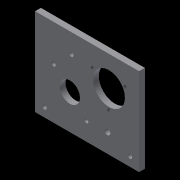
# Autodesk Inventor part: Main Outline
Saved by Autodesk Inventor 2014 SP1 (Build 180222100, 222)
## iProperties
Created: 2014-01-19
Part Number: Main Outline
Material: Generic
Document SubType Name: Modeling
Designer: Rauhul Varma
Density: 1 g/cm^3
Appearance: Default
Mass: 59.6414 g
Surface Area: 234.928 cm^2
Volume: 59.6414 cm^3
Author: Rauhul Varma
Autodesk Inventor part; units mm, degrees
ref_plane "YZ Plane" through (0, 0, 0) normal (1, 0, 0) x (0, 1, 0)
ref_plane "XZ Plane" through (0, 0, 0) normal (0, 1, 0) x (-1, 0, 0)
sketch "Sketch1" plane through (0, 0, 0) normal (0, 0, 1) x (1, 0, 0)
  line L0 (0, 0) -> (114.0582, 0)
  line L1 (114.0582, 0) -> (114.0582, 95.9104)
  line L2 (114.0582, 95.9104) -> (0, 95.9104)
  line L3 (0, 95.9104) -> (0, 0)
  line L4 (59.1, 17.1) -> (59.1, 59.1)
  line L5 (59.1, 59.1) -> (17.1, 59.1)
  line L6 (17.1, 59.1) -> (17.1, 17.1)
  line L7 (17.1, 17.1) -> (59.1, 17.1)
  line L8 (59.1, 17.1) -> (17.1, 59.1) construction
  line L9 (59.1, 59.1) -> (17.1, 17.1) construction
  circle A0 centre (38.1, 38.1) radius 38.1 construction
  circle A1 centre (38.1, 38.1) radius 20.2
  line L10 (45.4323, 38.1) -> (41.7662, 31.75)
  line L11 (41.7662, 31.75) -> (34.4338, 31.75)
  line L12 (34.4338, 31.75) -> (30.7677, 38.1)
  line L13 (30.7677, 38.1) -> (34.4338, 44.45)
  line L14 (34.4338, 44.45) -> (41.7662, 44.45)
  line L15 (41.7662, 44.45) -> (45.4323, 38.1)
  circle A2 centre (38.1, 38.1) radius 21.59 construction
  line L16 (38.1, 38.1) -> (81.0382, 62.8904) construction
  circle A3 centre (81.0382, 62.8904) radius 27.94 construction
  circle A4 centre (81.0382, 62.8904) radius 23.8125 construction
  circle A5 centre (81.0382, 62.8904) radius 17.4625
  circle A6 centre (38.1, 38.1) radius 14.2875
  line L17 (85.0105, 18.6054) -> (38.1, 38.1) construction
  circle A7 centre (81.0382, 62.8904) radius 33.02 construction
  circle A8 centre (38.1, 38.1) radius 25.4 construction
  circle A9 centre (38.1, 38.1) radius 11.1125
  line L18 (81.0382, 62.8904) -> (81.0382, 42.1545)
  circle A10 centre (81.0382, 42.1545) radius 2.0828 construction
  circle A11 centre (39.5622, 74.901) radius 10.16
  circle A12 centre (39.5622, 74.901) radius 6.35
  circle A13 centre (81.0382, 42.1545) radius 6.35 construction
  circle A14 centre (38.1, 38.1) radius 26.67 construction
  line L19 (85.0105, 18.6054) -> (87.4474, 24.4692)
  line L20 (85.0105, 18.6054) -> (82.5737, 12.7416)
  line L21 (87.4474, 24.4692) -> (77.6267, 28.5504)
  line L22 (82.5737, 12.7416) -> (72.2567, 17.029)
  circle A15 centre (103.8982, 10.16) radius 10.16
  circle A16 centre (103.8982, 10.16) radius 6.35
  circle A17 centre (10.16, 10.16) radius 10.16
  circle A18 centre (38.1, 38.1) radius 32.258 construction
  circle A19 centre (10.16, 10.16) radius 6.35
  point P0 (20.1395, 56.0605)
  point P1 (56.0605, 20.1395)
  point P2 (81.0382, 44.2373)
  point P3 (81.0382, 45.4279)
  point P4 (98.9961, 73.2584)
  point P5 (63.0804, 73.2584)
  point P6 (81.0382, 48.5045)
  point P7 (79.1467, 21.0422)
  dimension "d10" = 34.925
  dimension "d17" = 4.1656
  dimension "d25" = 12.7
  dimension "d0" = 42
  dimension "d1" = 42
  dimension "d2" = 76.2
  dimension "d3" = 40.4
  dimension "d4" = 12.7
  dimension "d5" = 43.18
  dimension "d6" = 55.88
  dimension "d7" = 49.5808
  dimension "d8" = 47.625
  dimension "d11" = 28.575
  dimension "d13" = 30
  dimension "d14" = 5.08
  dimension "d15" = 50.8
  dimension "d16" = 22.225
  dimension "d18" = 1.1906
  dimension "d21" = 360
  dimension "d23" = 20.32
  dimension "d24" = 12.7
  dimension "d26" = 3.0766
  dimension "d30" = 5.08
  dimension "d33" = 50.8
  dimension "d34" = 6.35
  dimension "d35" = 6.35
  dimension "d36" = 20.32
  dimension "d37" = 64.516
  dimension "d38" = 12.7
  constraints: 46 end point, 19 coincident, 17 centre point, 11 tangent, 6 point on line, 5 parallel, 5 perpendicular, 4 midpoint, 3 horizontal, 3 vertical alignment, 2 equal radius, 2 point on circle, 1 collinear, 1 line through centre, 1 symmetric about line, 23 other
  measures "d0" distance of L6.end L5.end
  measures "d1" distance of L5.end L4.end
  measures "d2" diameter of A0
  measures "d3" diameter of A1
  measures "d4" distance between parallel lines of L11 L14
  measures "d5" diameter of A2
  measures "d6" diameter of A3
  measures "d7" distance of L16.start L16.end
  measures "d8" diameter of A4
  measures "d11" diameter of A6
  measures "d13" angle of L0 L16
  measures "d14" radial gap between concentric circles of A7 A3
  measures "d15" diameter of A8
  measures "d16" diameter of A9
  measures "d18" distance of point (81.038, 44.237) point (81.038, 45.428)
  measures "d23" diameter of A11
  measures "d24" diameter of A12
  measures "d26" distance of point (81.038, 48.504) point (81.038, 45.428)
  measures "d30" radial gap between concentric circles of A2 A14
  measures "d33" distance of L17.start L17.end
  measures "d34" distance of L17.start L19.end
  measures "d35" distance from line of L20 point (79.147, 21.042)
  measures "d36" diameter of A17
  measures "d37" diameter of A18
  measures "d38" diameter of A19
ref_plane "Work Plane1" through (0, 0, -6.35) normal (0, 0, 1) x (1, 0, 0)
ref_plane "Work Plane2" through (0, 0, -41.875) normal (0, 0, 1) x (1, 0, 0)
ref_plane "Work Plane3" through (0, 0, -35.525) normal (0, 0, 1) x (1, 0, 0)
ref_plane "Work Plane4" through (0, 0, -92.675) normal (0, 0, 1) x (1, 0, 0)
ref_plane "Work Plane5" through (0, 0, -99.025) normal (0, 0, 1) x (1, 0, 0)
sketch "Sketch2" plane through (0, 0, -6.35) normal (0, 0, 1) x (1, 0, 0)
  line L0 (114.0582, 95.9104) -> (0, 95.9104) projected
  line L1 (0, 95.9104) -> (0, 0) projected
  line L2 (0, 0) -> (114.0582, 0) projected
  line L3 (114.0582, 0) -> (114.0582, 95.9104) projected
  circle A0 centre (81.0382, 62.8904) radius 17.4625 projected
  circle A1 centre (38.1, 38.1) radius 11.1125 projected
sketch "Sketch3" plane through (0, 0, -41.875) normal (0, 0, 1) x (1, 0, 0)
  line L0 (114.0582, 95.9104) -> (0, 95.9104) projected
  line L1 (114.0582, 0) -> (114.0582, 95.9104) projected
  circle A0 centre (81.0382, 62.8904) radius 17.4625 projected
  line L2 (0, 0) -> (114.0582, 0) projected
  line L3 (0, 95.9104) -> (0, 0) projected
  circle A1 centre (38.1, 38.1) radius 14.2875 projected
sketch "Sketch4" plane through (0, 0, -35.525) normal (0, 0, 1) x (1, 0, 0)
  line L0 (114.0582, 95.9104) -> (0, 95.9104) projected
  line L1 (0, 95.9104) -> (0, 0) projected
  line L2 (0, 0) -> (114.0582, 0) projected
  line L3 (114.0582, 0) -> (114.0582, 95.9104) projected
  circle A0 centre (81.0382, 62.8904) radius 17.4625 projected
  circle A1 centre (38.1, 38.1) radius 14.2875 projected
sketch "Sketch5" plane through (0, 0, -92.675) normal (0, 0, 1) x (1, 0, 0)
  line L0 (0, 95.9104) -> (0, 0) projected
  line L1 (114.0582, 95.9104) -> (0, 95.9104) projected
  line L2 (0, 0) -> (114.0582, 0) projected
  line L3 (114.0582, 0) -> (114.0582, 95.9104) projected
  circle A0 centre (81.0382, 62.8904) radius 17.4625 projected
sketch "Sketch6" plane through (0, 0, -99.025) normal (0, 0, 1) x (1, 0, 0)
  line L0 (0, 95.9104) -> (0, 0) projected
  line L1 (0, 0) -> (114.0582, 0) projected
  line L2 (114.0582, 0) -> (114.0582, 95.9104) projected
  line L3 (114.0582, 95.9104) -> (0, 95.9104) projected
  circle A0 centre (81.0382, 62.8904) radius 17.4625 projected
extrude "Extrusion1" add sketch "Sketch1" along normal blind 6.35 contours L3 A17 L0 | A17 L7 L4 L5 L6 L3 L2 L1 A15 L0 | A17 L6 L7 | A15 L1 L0 | A15 | A17 L7 L6 | L6 L5 L4 L7 A17 | A1 | A6 | A11 | A12 | A16 | A19
hole "Hole1" at (39.5622, 74.901, 0) at (10.16, 10.16, 0) at (103.8982, 10.16, 0) direction (0, 0, 1) diameter 4.9784 end through all clearance for "Flat Head Machine Screw (82)" size "#10" standard "Ansi Unified Screw Threads"
hole "Hole2" at (81.0382, 42.1545, 0) at (98.9961, 73.2584, 0) at (63.0804, 73.2584, 0) direction (0, 0, 1) diameter 3.9624 end through all thread size "10-32 UNF" class "2B" standard "ANSI Unified Screw Threads"
hole "Hole3" at (79.1467, 21.0422, 0) direction (0, 0, 1) diameter 6.5278 end through all clearance for "Flat Head Machine Screw (82)" size "1/4" standard "Ansi Unified Screw Threads"
hole "Hole4" at (20.1395, 56.0605, 0) at (56.0605, 20.1395, 0) direction (0, 0, 1) diameter 4.9784 end through all countersink diameter 10.795 countersink angle 82 clearance for "Flat Head Machine Screw (82)" size "#10" standard "Ansi Unified Screw Threads"
equation "\"d30\" = d14"
body "Solid1"
